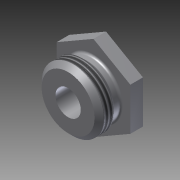
# Autodesk Inventor part: Деталь10000
Saved by Autodesk Inventor 2012 SP2 (Build 160219200, 219)
## iProperties
Created: 2014-03-31
Part Number: Деталь10000
Material: Default
Document SubType Name: Modeling
Designer: N750
Density: 1 g/cm^3
Author: N750
Autodesk Inventor part; units mm, degrees
ref_plane "YZ Plane" through (0, 0, 0) normal (1, 0, 0) x (0, 1, 0)
ref_plane "XZ Plane" through (0, 0, 0) normal (0, 1, 0) x (-1, 0, 0)
ref_plane "XY Plane" through (0, 0, 0) normal (0, 0, 1) x (1, 0, 0)
sketch "Эскиз1" plane through (0, 0, 0) normal (0, 0, 1) x (1, 0, 0)
  point P0 (0, 0)
sketch "Эскиз2" plane through (0, 0, 0) normal (0, 1, 0) x (-1, 0, 0)
  line L0 (0, 18.4752) -> (16, 9.2376)
  line L1 (16, 9.2376) -> (16, -9.2376)
  line L2 (16, -9.2376) -> (0, -18.4752)
  line L3 (0, -18.4752) -> (-16, -9.2376)
  line L4 (-16, -9.2376) -> (-16, 9.2376)
  line L5 (-16, 9.2376) -> (0, 18.4752)
  circle A0 centre (0, 0) radius 5.5
  dimension "d0" = 32
  dimension "d1" = 11
  constraints: 12 end point, 2 coincident, 1 centre point, 14 other
  measures "d0" distance of L3.end L1.end
  measures "d1" diameter of A0
extrude "Выдавливание1" add sketch "Эскиз2" along normal blind 5.5
sketch "Эскиз3" plane through (0, 5.5, 0) normal (0, 1, 0) x (1, 0, 0)
  circle A0 centre (0, 0) radius 5.5 projected
  circle A1 centre (0, 0) radius 10
  dimension "d4" = 20
  constraints: 1 centre point, 1 coincident
  measures "d4" diameter of A1
extrude "Выдавливание2" add sketch "Эскиз3" along normal blind 2.5
chamfer "Фаска1" distance 1 angle 45 1 edges at (-10, 8, 0) measured on face at (8.3499, 8, 1.2365)
sketch "Эскиз4" plane through (0, 0, 0) normal (0, -1, 0) x (1, 0, 0)
  circle A0 centre (0, 0) radius 5.5 projected
  circle A1 centre (0, 0) radius 11.75
  dimension "d10" = 23.5
  constraints: 1 centre point, 1 coincident
  measures "d10" diameter of A1
extrude "Выдавливание3" add sketch "Эскиз4" along normal blind 3
sketch "Эскиз5" plane through (0, -3, 0) normal (0, -1, 0) x (1, 0, 0)
  circle A0 centre (0, 0) radius 11.75 projected
  circle A1 centre (0, 0) radius 13.5
  dimension "d13" = 27
  constraints: 1 centre point, 1 coincident
  measures "d13" diameter of A1
extrude "Выдавливание4" add sketch "Эскиз5" along normal blind 8
sketch "Эскиз6" plane through (0, -3, 0) normal (0, -1, 0) x (1, 0, 0)
  circle A0 centre (0, 0) radius 5.5 projected
  circle A1 centre (0, 0) radius 11.75 projected
extrude "Выдавливание5" add sketch "Эскиз6" along normal blind 8
thread "Резьба1" size "G 3/4-14" class "A" standard "BSP Pipe Threads" full length
chamfer "Фаска2" distance 2 angle 45 1 edges at (-13.5, -11, 0) measured on face at (12.6721, -11, -2.0142)
chamfer "Фаска3" distance 1.75 angle 45 1 edges at (-13.5, -3, 0)
fillet "Сопряжение1" radius 0.5 2 edges at (-11.7501, -3, 0) (-11.75, -3, 0)
fillet "Сопряжение2" radius 1 1 edges at (-11.75, 0, 0)
